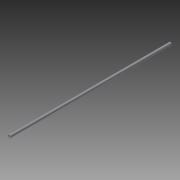
# Autodesk Inventor part: GE-13057
Saved by Autodesk Inventor 2013 (Build 170138000, 138)
## iProperties
Created: 2013-01-03
Part Number: GE-13057
Material: Generic
Document SubType Name: Modeling
Designer: Phillip
Density: 1 g/cm^3
Author: Phillip
Autodesk Inventor part; units mm, degrees
ref_plane "YZ Plane" through (0, 0, 0) normal (1, 0, 0) x (0, 1, 0)
ref_plane "XY Plane" through (0, 0, 0) normal (0, 0, 1) x (1, 0, 0)
sketch "Sketch1" plane through (0, 0, 0) normal (0, 0, 1) x (1, 0, 0)
  circle A0 centre (0, 0) radius 8.5725
  circle A1 centre (0, 0) radius 6.2611
  dimension "d0" = 17.145
  dimension "d2" = 2.3114
  constraints: 2 centre point, 2 coincident
  measures "d0" diameter of A0
  measures "d2" radial gap between concentric circles of A0 A1
extrude "Extrusion1" add sketch "Sketch1" against normal blind 1009.65
ref_plane "Work Plane1" through (0, 8.5725, 0) normal (0, 1, 0) x (-1, 0, 0)
body "Solid1"
